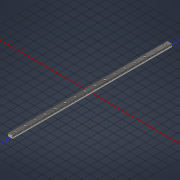
# Autodesk Inventor part: MGN12H Linear-Rail (400mm)
Saved by Autodesk Inventor 2022.2 (Build 262287010, 287A)
## iProperties
Created: 2022-03-15
Part Number: MGN12H Linear-Rail (400mm)
Material: Stahl, hochfest, niedrig legiert
Document SubType Name: Modeling
Designer: sleib
Density: 7.85 g/cm^3
Appearance: Stahl - poliert
Author: sleib
Autodesk Inventor part; units mm, degrees
ref_plane "YZ Plane" through (0, 0, 0) normal (1, 0, 0) x (0, 1, 0)
ref_plane "XZ Plane" through (0, 0, 0) normal (0, 1, 0) x (-1, 0, 0)
ref_plane "XY Plane" through (0, 0, 0) normal (0, 0, 1) x (1, 0, 0)
sketch "Skizze1" plane through (0, 0, 0) normal (0, 0, 1) x (1, 0, 0)
  line L0 (5.5, 0) -> (-5.5, 0)
  line L1 (6, 0.5) -> (5.5, 0)
  line L2 (6, 4.1421) -> (6, 0.5)
  arc A0 (6, 4.1421) -> (5.8448, 4.3734) centre (5.75, 4.1421) ccw
  arc A1 (5.2672, 4.8727) -> (5.8448, 4.3734) centre (6.3, 5.4838) ccw
  arc A2 (5.2672, 4.8727) -> (5.0738, 4.9945) centre (5.052, 4.7454) ccw
  line L3 (4.7277, 5.0248) -> (5.0738, 4.9945)
  arc A3 (4.5, 5.2576) -> (4.7277, 5.0248) centre (4.7495, 5.2738) ccw
  line L4 (4.5, 5.7099) -> (4.5, 5.2576)
  arc A4 (4.7287, 5.9753) -> (4.5, 5.7099) centre (4.7495, 5.7262) ccw
  line L5 (5.0948, 6.0073) -> (4.7287, 5.9753)
  arc A5 (5.0948, 6.0073) -> (5.2845, 6.1232) centre (5.073, 6.2564) ccw
  arc A6 (5.8448, 6.5941) -> (5.2845, 6.1232) centre (6.3, 5.4838) ccw
  arc A7 (5.8448, 6.5941) -> (6, 6.8254) centre (5.75, 6.8254) ccw
  line L6 (6, 7.5) -> (6, 6.8254)
  line L7 (5.5, 8) -> (6, 7.5)
  line L8 (-5.5, 8) -> (5.5, 8)
  line L9 (-6, 7.5) -> (-5.5, 8)
  line L10 (-6, 6.8254) -> (-6, 7.5)
  arc A8 (-6, 6.8254) -> (-5.8448, 6.5941) centre (-5.75, 6.8254) ccw
  arc A9 (-5.2845, 6.1232) -> (-5.8448, 6.5941) centre (-6.3, 5.4838) ccw
  arc A10 (-5.2845, 6.1232) -> (-5.0948, 6.0073) centre (-5.073, 6.2564) ccw
  line L11 (-4.7287, 5.9753) -> (-5.0948, 6.0073)
  arc A11 (-4.5, 5.7099) -> (-4.7287, 5.9753) centre (-4.7495, 5.7262) ccw
  line L12 (-4.5, 5.2576) -> (-4.5, 5.7099)
  arc A12 (-4.7277, 5.0248) -> (-4.5, 5.2576) centre (-4.7495, 5.2738) ccw
  line L13 (-5.0738, 4.9945) -> (-4.7277, 5.0248)
  arc A13 (-5.0738, 4.9945) -> (-5.2672, 4.8727) centre (-5.052, 4.7454) ccw
  arc A14 (-5.8448, 4.3734) -> (-5.2672, 4.8727) centre (-6.3, 5.4838) ccw
  arc A15 (-5.8448, 4.3734) -> (-6, 4.1421) centre (-5.75, 4.1421) ccw
  line L14 (-6, 0.5) -> (-6, 4.1421)
  line L15 (-5.5, 0) -> (-6, 0.5)
  line L16 (-10.5, 0) -> (10.5, 0) construction
  line L17 (0, -1.6) -> (0, 9.6) construction
  circle A16 centre (-6.3, 5.4838) radius 1.2 construction
  circle A17 centre (6.3, 5.4838) radius 1.2 construction
  line L18 (-4.7287, 5.9753) -> (-5.2259, 6.0188) construction
  line L19 (-4.7277, 5.0248) -> (-5.2097, 4.9826) construction
  point P0 (0, 0)
  point P1 (0, 0)
  point P2 (10.5, 0)
  point P3 (0, -1.6)
  point P4 (0, 8)
  point P5 (-4.9008, 5.0096)
  point P6 (-4.9118, 5.9913)
  point P7 (-4.5, 5.4838)
  dimension "d0" = 8
  dimension "d1" = 12
  dimension "d3" = 1.2
  dimension "d4" = 0.25
  dimension "d5" = 0.25
  dimension "d6" = 0.25
  dimension "d7" = 0.25
  dimension "d8" = 1.2
  dimension "d10" = 9
  dimension "d11" = 0.5
  dimension "d12" = 0.5
  dimension "d13" = 0.5
  dimension "d14" = 0.5
  dimension "d16" = 5.4838
  dimension "d17" = 12.6
  dimension "d18" = 10
  dimension "d21" = 0.9817
  dimension "d24" = 0.4523
  dimension "d25" = 1.5109
  dimension "d26" = 0.948
  dimension "d27" = 1.2505
  dimension "d28" = 0.25
  constraints: 36 end point, 34 point on circle, 18 centre point, 9 tangent, 8 equal radius, 5 midpoint, 3 collinear, 3 parallel, 2 coincident, 2 concentric, 2 equal length, 2 perpendicular, 2 vertical alignment, 1 horizontal alignment, 1 vertical, 3 other
  measures "d0" distance between parallel lines of L0 L8
  measures "d1" distance between parallel lines of L2 L14
  measures "d3" radius of A14
  measures "d4" radius of A13
  measures "d5" radius of A12
  measures "d6" radius of A11
  measures "d7" radius of A10
  measures "d8" radius of A9
  measures "d10" distance between parallel lines of L4 L12
  measures "d11" horizontal distance of L14.start L15.start
  measures "d12" horizontal distance of L14.start L15.start
  measures "d13" horizontal distance of L9.end L10.end
  measures "d14" horizontal distance of L9.end L10.end
  measures "d16" distance from line of A9.centre L0
  measures "d17" distance of A6.centre A14.centre
  measures "d18" angle of L13 L11
  measures "d21" vertical distance of point (-4.901, 5.01) point (-4.912, 5.991)
  measures "d24" distance of A12.centre A11.centre
  measures "d25" vertical distance of A13.centre A10.centre
  measures "d26" distance from line of A13.centre L14
  measures "d27" distance from line of A12.centre L14
  measures "d28" radius of A15
extrude "Extrusion1" add sketch "Skizze1" along normal mid plane 400
sketch "Skizze2" plane through (-5.5, 8, 200) normal (0, 1, 0) x (1, 0, 0)
  line L0 (0, 400) -> (0, 0) projected
  line L1 (11, 0) -> (0, 0) projected
  line L2 (11, 400) -> (11, 0) projected
  line L3 (0, 400) -> (11, 400) projected
  line L4 (0, 0) -> (11, 0) projected
  line L5 (5.5, 0) -> (5.5, 400) construction
  line L6 (0, 400) -> (11, 400) projected
  point P0 (5.5, 200)
  point P1 (5.5, 12.5)
  point P2 (5.5, 37.5)
  point P3 (5.5, 62.5)
  point P4 (5.5, 87.5)
  point P5 (5.5, 112.5)
  point P6 (5.5, 137.5)
  point P7 (5.5, 162.5)
  point P8 (5.5, 187.5)
  point P9 (5.5, 212.5)
  point P10 (5.5, 237.5)
  point P11 (5.5, 262.5)
  point P12 (5.5, 287.5)
  point P13 (5.5, 312.5)
  point P14 (5.5, 337.5)
  point P15 (5.5, 362.5)
  point P16 (5.5, 387.5)
  dimension "d31" = 12.5
  dimension "d34" = 25
  constraints: 2 end point, 2 midpoint, 1 point on line, 1 vertical, 15 other
  measures "d31" distance from line of point (5.5, 12.5) L1
  measures "d34" distance of point (5.5, 12.5) point (5.5, 37.5)
hole "Bohrung1" at (0, 8, 187.5) at (0, 8, 162.5) at (0, 8, 137.5) at (0, 8, 112.5) at (0, 8, 87.5) at (0, 8, 62.5) at (0, 8, 37.5) at (0, 8, 12.5) at (0, 8, -12.5) at (0, 8, -37.5) at (0, 8, -62.5) at (0, 8, -87.5) at (0, 8, -112.5) at (0, 8, -137.5) at (0, 8, -162.5) at (0, 8, -187.5) direction (0, -1, 0) diameter 3.4 end through all counterbore diameter 6 counterbore depth 3.4 clearance for "Inbusschraube DIN EN ISO 4762" size "M3" standard "DIN"
chamfer "Fase1" distance 0.5 angle 45 16 edges at (0, 8, 184.5) (0, 8, 159.5) (0, 8, 134.5) (0, 8, 109.5) (0, 8, 84.5) (0, 8, 59.5) (0, 8, 34.5) (0, 8, 9.5) (0, 8, -15.5) (0, 8, -40.5) (0, 8, -65.5) (0, 8, -90.5) (0, 8, -115.5) (0, 8, -140.5) (0, 8, -165.5) (0, 8, -190.5)
